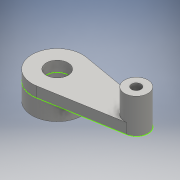
# Autodesk Inventor part: 240510_3Dsketch02
Saved by Autodesk Inventor 2016 (Build 200138000, 138)
## iProperties
Created: 2024-05-10
Part Number: 240510_3Dsketch02
Material: 일반
Document SubType Name: Modeling
Designer: pc
Density: 1 g/cm^3
Appearance: 기본값
Author: pc
Autodesk Inventor part; units mm, degrees
ref_plane "YZ Plane" through (0, 0, 0) normal (1, 0, 0) x (0, 1, 0)
ref_plane "XZ Plane" through (0, 0, 0) normal (0, 1, 0) x (-1, 0, 0)
ref_plane "XY Plane" through (0, 0, 0) normal (0, 0, 1) x (1, 0, 0)
sketch "스케치1" plane through (0, 0, 0) normal (0, 0, 1) x (1, 0, 0)
  circle A0 centre (-12.5044, 1.9437) radius 3.1513
  arc A1 (-11.264, 9.1039) -> (-11.264, -5.2166) centre (-12.5044, 1.9437) ccw
  circle A2 centre (10.3031, 1.9437) radius 3.3737
  line L0 (-11.264, 9.1039) -> (10.879, 5.2678)
  line L1 (-11.264, -5.2166) -> (10.879, -1.3805)
  circle A3 centre (10.3031, 1.9437) radius 1.3624
  point P0 (0, 0)
  constraints: 4 centre point, 4 end point, 4 point on circle, 4 tangent, 2 coincident
extrude "돌출1" add sketch "스케치1" along normal blind 3 contours L0 A2 L1 A1
extrude "돌출2" add sketch "스케치1" along normal blind 10 contours A2
sketch "스케치2" plane through (0, 0, 0) normal (0, 0, -1) x (-1, 0, 0)
  circle A0 centre (12.4874, 1.9523) radius 7.2656
  circle A1 centre (12.4874, 1.9523) radius 3.17
  point P0 (0, 0)
  constraints: 2 centre point, 1 coincident
extrude "돌출3" add sketch "스케치2" along normal blind 5
